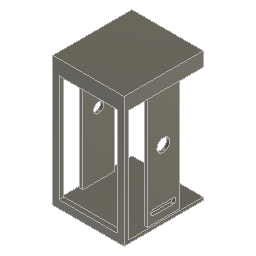
Spool Stand (Autodesk Fusion 360 design; units mm, degrees)
part number: 2026-02-26-14-15-08-789
Autodesk Fusion 360 part; units mm, degrees
sketch "Sketch1" plane through (0, 0, 0) normal (0, 0, 1) x (1, 0, 0)
  line L0 (0, 20) -> (45, 20)
  line L1 (45, 20) -> (45, -30)
  line L2 (45, -30) -> (0, -30)
  line L3 (0, -30) -> (0, 20)
  dimension "d1" = 50
  dimension "d2" = 45
  constraint horizontal L0
  constraint vertical L1
  constraint horizontal L2
  constraint vertical L3
  measures "d1" distance of L0.start L2.end
  measures "d2" distance of L0.start L0.end
extrude "Extrude1" add sketch "Sketch1" along normal blind 2
sketch "Sketch2" plane through (0, 0, 2) normal (0, 0, 1) x (-1, 0, 0)
  line L0 (0, 30) -> (-45, 30)
  line L1 (-45, 30) -> (-45, -20)
  line L2 (-45, -20) -> (0, -20)
  line L3 (0, -20) -> (0, 30)
  line L4 (-1, -6) -> (-3, -6)
  line L5 (-3, -6) -> (-3, 14)
  line L6 (-3, 14) -> (-1, 14)
  line L7 (-1, 14) -> (-1, -6)
  line L8 (-42, -5.8571) -> (-44, -5.8571)
  line L9 (-44, -5.8571) -> (-44, 14.1429)
  line L10 (-44, 14.1429) -> (-42, 14.1429)
  line L11 (-42, 14.1429) -> (-42, -5.8571)
  line L12 (-45, -20) -> (-45, 30)
  line L13 (0, 27) -> (-45, 27)
  line L14 (-45, 27) -> (-45, 30)
  line L15 (-45, 30) -> (0, 30)
  line L16 (0, 30) -> (0, 27)
  dimension "d5" = 20
  dimension "d6" = 2
  dimension "d10" = 2
  dimension "d11" = 39
  dimension "d44" = 1
  constraint horizontal L4
  constraint vertical L5
  constraint horizontal L6
  constraint vertical L7
  constraint horizontal L8
  constraint vertical L9
  constraint horizontal L10
  constraint vertical L11
  constraint equal L5 L11
  constraint horizontal L13
  constraint vertical L14
  constraint horizontal L15
  constraint vertical L16
  constraint coincident L0.end L1.start
  constraint coincident L3 L13.start
  measures "d5" distance of L4.start L6.end
  measures "d6" distance of L4.start L4.end
  measures "d10" distance of L8.start L8.end
  measures "d11" distance of L5 L11
  measures "d44" distance of L9 L12
extrude "Extrude2" add sketch "Sketch2" along normal blind 50 contours L4 L5 L6 L7 | L8 L9 L10 L11
sketch "Sketch3" plane through (42, 0, 0) normal (-1, 0, 0) x (0, -1, 0)
  line L0 (-5.8571, 2) -> (14.1429, 2)
  line L1 (14.1429, 2) -> (14.1429, 52)
  line L2 (14.1429, 52) -> (-5.8571, 52)
  line L3 (-5.8571, 52) -> (-5.8571, 2)
  circle A0 centre (4.1429, 42) radius 4.1125
  dimension "d15" = 8.225
  dimension "d16" = 40
  dimension "d34" = 10
  measures "d15" diameter of A0
  measures "d16" distance of L0 A0.centre
  measures "d34" distance of L1 A0.centre
extrude "Extrude3" cut sketch "Sketch3" against normal blind 2 contours A0
sketch "Sketch4" plane through (1, 0, 0) normal (-1, 0, 0) x (0, -1, 0)
  line L0 (-6, 2) -> (14, 2)
  line L1 (14, 2) -> (14, 52)
  line L2 (14, 52) -> (-6, 52)
  line L3 (-6, 52) -> (-6, 2)
  circle A0 centre (4, 42) radius 3.25
  dimension "d19" = 6.5
  dimension "d33" = 10
  dimension "d41" = 10
  measures "d19" diameter of A0
  measures "d33" distance of L1 A0.centre
  measures "d41" distance of L2 A0.centre
extrude "Extrude4" cut sketch "Sketch4" against normal blind 2 contours A0
extrude "Extrude5" add sketch "Sketch2" along normal blind 80 contours L0 L1 L3 L12 L13 L14 L15 L16
sketch "Sketch6" plane through (0, -30, 0) normal (0, -1, 0) x (1, 0, 0)
  line L0 (0, 0) -> (45, 0)
  line L1 (45, 0) -> (45, 82)
  line L2 (0, 82) -> (0, 0)
  line L3 (4, 79) -> (41, 79)
  line L4 (41, 79) -> (41, 5)
  line L5 (41, 5) -> (4, 5)
  line L6 (4, 5) -> (4, 79)
  line L7 (45, 82) -> (0, 82)
  dimension "d49" = 74
  dimension "d50" = 5
  dimension "d63" = 37
  dimension "d64" = 4
  constraint horizontal L3
  constraint vertical L4
  constraint horizontal L5
  constraint vertical L6
  measures "d49" distance of L3.end L4.end
  measures "d50" distance of L0 L5
  measures "d63" distance of L4.end L5.end
  measures "d64" distance of L2 L6
extrude "Extrude6" cut sketch "Sketch6" against normal blind 3 contours L3 L4 L5 L6
extrude "Extrude9" add 1 faces at (16.3333, -29, 79) along direction (0, 0, -1) blind 1.25
extrude "Extrude10" add 2 faces at (43.3333, -0.8095, 52) (1.6667, -0.6667, 52) along direction (0, 0, 1) blind 26
sketch "Sketch9" plane through (0, -27, 0) normal (0, 1, 0) x (-1, 0, 0)
  line L0 (-45, 2) -> (0, 2)
  line L1 (0, 2) -> (0, 82)
  line L2 (0, 82) -> (-45, 82)
  line L3 (-45, 82) -> (-45, 2)
  line L4 (-45, 82) -> (0, 82)
  line L5 (0, 82) -> (0, 73)
  line L6 (0, 73) -> (-45, 73)
  line L7 (-45, 73) -> (-45, 82)
  line L8 (-41, 5) -> (-41, 77.75)
  line L9 (-41, 77.75) -> (-4, 77.75)
  line L10 (-4, 77.75) -> (-4, 5)
  line L11 (-4, 5) -> (-41, 5)
  dimension "d51" = 9
  constraint horizontal L4
  constraint vertical L5
  constraint horizontal L6
  constraint vertical L7
  constraint coincident L1 L5.end
  constraint coincident L2.end L3.start
  measures "d51" distance of L2.end L6.end
extrude "Extrude11" add sketch "Sketch9" along normal blind 37 contours L1 L2 L3 L4 L5 L6 L7 L8 L9 L10 | L6 L8 L9 L10
extrude "Extrude12" add 1 faces at (30, 10, 79) along direction (0, 1, 0) blind 5
sketch "Sketch10" plane through (0, 0, 73) normal (0, 0, -1) x (1, 0, 0)
  line L0 (1, -6) -> (1, 14)
  line L1 (1, 14) -> (3, 14)
  line L2 (3, 14) -> (3, -6)
  line L3 (3, -6) -> (1, -6)
  line L4 (42, -5.8571) -> (42, 14.1429)
  line L5 (42, 14.1429) -> (44, 14.1429)
  line L6 (44, 14.1429) -> (44, -5.8571)
  line L7 (44, -5.8571) -> (42, -5.8571)
  line L8 (4, 27) -> (0, 27)
  line L9 (0, 27) -> (0, -15)
  line L10 (0, -15) -> (45, -15)
  line L11 (45, -15) -> (45, 27)
  line L12 (40, -12.6) -> (5, -12.6)
  line L13 (5, -12.6) -> (5, 25)
  line L14 (5, 25) -> (40, 25)
  line L15 (40, 25) -> (40, -12.6)
  line L16 (45, 27) -> (41, 27)
  line L17 (41, 27) -> (4, 27)
  line L18 (40, 25) -> (5, 25)
  line L19 (5, 25) -> (5, 27)
  line L20 (5, 27) -> (40, 27)
  line L21 (40, 27) -> (40, 25)
  dimension "d74" = 2
  dimension "d75" = 37.6
  constraint horizontal L12
  constraint vertical L13
  constraint horizontal L14
  constraint vertical L15
  constraint horizontal L18
  constraint vertical L19
  constraint horizontal L20
  constraint vertical L21
  constraint coincident L17 L19.end
  measures "d74" distance of L14 L20
  measures "d75" distance of L12.start L14.end
extrude "Extrude13" cut sketch "Sketch10" against normal blind 8 contours L12 L13 L14 L15 L18
extrude "Extrude14" add 1 faces at (16.3333, -29, 77.75) along direction (0, 0, -1) blind 5
extrude "Extrude15" cut sketch "Sketch10" against normal blind 8 contours L14 L17 L18 L19 L20 L21
sketch "Sketch11" plane through (0, -27, 0) normal (0, 1, 0) x (-1, 0, 0)
  line L0 (-4, 72.75) -> (-4, 5)
  line L1 (-4, 5) -> (-41, 5)
  line L2 (-41, 5) -> (-41, 72.75)
  line L3 (-41, 72.75) -> (-4, 72.75)
  line L4 (0, 73) -> (-5, 73)
  line L5 (-5, 73) -> (-5, 81)
  line L6 (-5, 81) -> (-40, 81)
  line L7 (-40, 81) -> (-40, 73)
  line L8 (-40, 73) -> (-45, 73)
  line L9 (-45, 73) -> (-45, 2)
  line L10 (-45, 2) -> (0, 2)
  line L11 (0, 2) -> (0, 73)
  line L12 (-40, 74) -> (-5, 74)
  line L13 (-5, 74) -> (-5, 73)
  line L14 (-5, 73) -> (-40, 73)
  line L15 (-40, 73) -> (-40, 74)
  constraint horizontal L12
  constraint vertical L13
  constraint horizontal L14
  constraint vertical L15
  constraint coincident L4.end L5.start
  constraint coincident L7 L12.start
extrude "Extrude16" add sketch "Sketch11" along normal blind 3.5 contours L5 L7 L12 L13 L14 L15
sketch "Sketch12" plane through (44, 0, 0) normal (1, 0, 0) x (0, 1, 0)
  line L0 (5.8571, 73) -> (-14.1429, 73)
  line L1 (-14.1429, 73) -> (-14.1429, 2)
  line L2 (-14.1429, 2) -> (5.8571, 2)
  line L3 (5.8571, 2) -> (5.8571, 73)
  circle A0 centre (-4.1429, 42) radius 4.1125
  line L4 (-12.1429, 10) -> (3.8571, 10)
  line L5 (3.8571, 10) -> (3.8571, 6.5)
  line L6 (3.8571, 6.5) -> (-12.1429, 6.5)
  line L7 (-12.1429, 6.5) -> (-12.1429, 10)
  dimension "d65" = 3.5
  dimension "d66" = 2
  dimension "d67" = 16
  constraint horizontal L4
  constraint vertical L5
  constraint horizontal L6
  constraint vertical L7
  measures "d65" distance of L4.start L6.end
  measures "d66" distance of L3 L5
  measures "d67" distance of L4.start L4.end
extrude "Extrude17" cut sketch "Sketch12" against normal blind 2 contours L4 L5 L6 L7
fillet "Fillet1" radius 1.75 4 edges at (43, 3.8571, 6.5) (43, 3.8571, 10) (43, -12.1429, 10) (43, -12.1429, 6.5)
extrude "Extrude18" add 1 faces at (30, 15, 79) along direction (0, 1, 0) blind 5
sketch "Sketch13" plane through (0, 0, 73) normal (0, 0, -1) x (1, 0, 0)
  line L0 (40, 23.5) -> (40, -12.6)
  line L1 (40, -12.6) -> (5, -12.6)
  line L2 (5, -12.6) -> (5, 23.5)
  line L3 (5, 23.5) -> (40, 23.5)
  line L4 (45, 27) -> (0, 27)
  line L5 (0, 27) -> (0, -20)
  line L6 (0, -20) -> (45, -20)
  line L7 (45, -20) -> (45, 27)
  line L8 (1, -6) -> (1, 14)
  line L9 (1, 14) -> (3, 14)
  line L10 (3, 14) -> (3, -6)
  line L11 (3, -6) -> (1, -6)
  line L12 (42, -5.8571) -> (42, 14.1429)
  line L13 (42, 14.1429) -> (44, 14.1429)
  line L14 (44, 14.1429) -> (44, -5.8571)
  line L15 (44, -5.8571) -> (42, -5.8571)
  line L16 (40, -12.6) -> (5, -12.6)
  line L17 (5, -12.6) -> (5, -17)
  line L18 (5, -17) -> (40, -17)
  line L19 (40, -17) -> (40, -12.6)
  constraint horizontal L16
  constraint vertical L17
  constraint horizontal L18
  constraint vertical L19
  constraint coincident L0.end L1.start
extrude "Extrude19" cut sketch "Sketch13" against normal blind 8 contours L1 L16 L17 L18 L19
